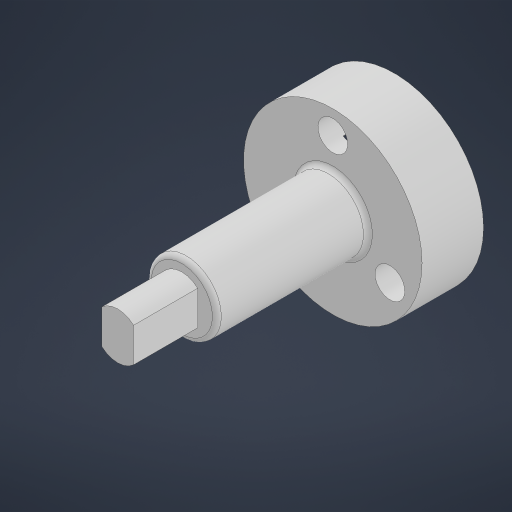
# Autodesk Inventor part: Mounting Adapter
Saved by Autodesk Inventor 2023 (Build 270158000, 158)
## iProperties
Created: 2023-03-26
Part Number: Mounting Adapter
Material: Generic
Document SubType Name: Modeling
Designer: Michael
Density: 1 g/cm^3
Appearance: Default
Author: Michael
Autodesk Inventor part; units mm, degrees
ref_plane "YZ Plane" through (0, 0, 0) normal (1, 0, 0) x (0, 1, 0)
ref_plane "XZ Plane" through (0, 0, 0) normal (0, 1, 0) x (-1, 0, 0)
ref_plane "XY Plane" through (0, 0, 0) normal (0, 0, 1) x (1, 0, 0)
sketch "Sketch1" plane through (0, 0, 0) normal (0, 0, 1) x (1, 0, 0)
  line L0 (6.5, 0) -> (19.5, 0) construction
  line L1 (0, 0) -> (13, 0)
  line L2 (13, 0) -> (6.5, 11.2583)
  line L3 (0, 0) -> (6.5, 11.2583)
  circle A0 centre (6.5, 3.7528) radius 6
  line L4 (6.5, 11.2583) -> (6.5, 0)
  circle A1 centre (6.5, 11.2583) radius 1.7
  circle A2 centre (13, 0) radius 1.7
  circle A3 centre (0, 0) radius 1.7
  circle A4 centre (6.5, 3.7528) radius 10.16
  point P0 (1.7, 0)
  point P1 (0.85, 1.4722)
  point P2 (0.9092, 1.5748)
  point P3 (5.5908, 9.6835)
  point P4 (5.65, 9.7861)
  point P5 (7.35, 9.7861)
  point P6 (7.4092, 9.6835)
  point P7 (12.0908, 1.5748)
  point P8 (12.15, 1.4722)
  point P9 (11.3, 0)
  point P10 (11.1815, 0)
  point P11 (1.8185, 0)
  dimension "d6" = 13
  dimension "d7" = 13
  dimension "d8" = 13
  dimension "d9" = 12
  dimension "d10" = 3.4
  dimension "d11" = 3.4
  dimension "d12" = 3.4
  dimension "d13" = 20.32
  constraints: 10 end point, 5 centre point, 4 coincident, 1 horizontal, 1 midpoint, 1 perpendicular, 1 point on line
  measures "d6" distance of L1.start L1.end
  measures "d7" distance of L1.end L2.end
  measures "d8" distance of L2.end L1.start
  measures "d9" diameter of A0
  measures "d10" diameter of A1
  measures "d11" diameter of A2
  measures "d12" diameter of A3
  measures "d13" diameter of A4
extrude "Extrusion1" add sketch "Sketch1" along normal blind 5
sketch "Sketch2" plane through (6.5, 3.7528, 5) normal (0, 0, 1) x (1, 0, 0)
  arc A0 (5.5908, -2.1779) -> (0.9092, 5.9307) centre (0, 0) ccw projected
  circle A1 centre (0, 0) radius 6
  circle A2 centre (0, 0) radius 3
  circle A3 centre (0, 0) radius 10.16 projected
  arc A4 (-5.65, -2.2805) -> (-4.8, -3.7528) centre (-6.5, -3.7528) ccw projected
  line L0 (-5.65, -2.2805) -> (-5.5908, -2.1779) projected
  arc A5 (-0.9092, 5.9307) -> (-5.5908, -2.1779) centre (0, 0) ccw projected
  line L1 (-0.9092, 5.9307) -> (-0.85, 6.0333) projected
  arc A6 (0.85, 6.0333) -> (-0.85, 6.0333) centre (0, 7.5056) ccw projected
  line L2 (0.85, 6.0333) -> (0.9092, 5.9307) projected
  arc A7 (5.5908, -2.1779) -> (0.9092, 5.9307) centre (0, 0) ccw projected
  line L3 (5.5908, -2.1779) -> (5.65, -2.2805) projected
  arc A8 (4.8, -3.7528) -> (5.65, -2.2805) centre (6.5, -3.7528) ccw projected
  line L4 (4.8, -3.7528) -> (4.6815, -3.7528) projected
  arc A9 (-4.6815, -3.7528) -> (4.6815, -3.7528) centre (0, 0) ccw projected
  line L5 (-4.6815, -3.7528) -> (-4.8, -3.7528) projected
  circle A10 centre (0, 7.5056) radius 1.7
  circle A11 centre (-6.5, -3.7528) radius 1.7
  circle A12 centre (6.5, -3.7528) radius 1.7
  point P0 (0.9092, 5.9307)
  point P1 (0.9092, 5.9307)
  point P2 (-4.6815, -3.7528)
  point P3 (-5.65, -2.2805)
  dimension "d16" = 6
  constraints: 5 coincident, 3 centre point, 6 other
  measures "d16" diameter of A2
extrude "Extrusion2" add sketch "Sketch2" along normal blind 2 contours A1 A12 A11 A10 A0 | L3 A12 A1 | A1 A10 L2 | A12 L4 A1 | A1 L1 A10 | L5 A11 A1 | A1 A11 L0 | A2 | A3
sketch "Sketch3" plane through (6.5, 3.7528, 7) normal (0, 0, 1) x (1, 0, 0)
  circle A0 centre (0, 0) radius 4
  point P0 (-6.5, -3.7528)
  dimension "d19" = 8
  constraints: 1 centre point
  measures "d19" diameter of A0
extrude "Extrusion3" add sketch "Sketch3" along normal blind 17
sketch "Sketch5" plane through (6.5, 3.7528, 24) normal (0, 0, 1) x (1, 0, 0)
  circle A0 centre (0, 0) radius 2
  point P0 (-6.5, -3.7528)
  dimension "d22" = 4
  constraints: 1 centre point
  measures "d22" diameter of A0
extrude "Extrusion4" cut sketch "Sketch5" against normal blind 22.6875
sketch "Sketch7" plane through (6.5, 3.7528, 24) normal (0, 0, 1) x (1, 0, 0)
  arc A0 (1.85, 1.9666) -> (-1.85, 1.9666) centre (0, 0) ccw
  line L0 (-1.85, 1.9666) -> (-1.85, -1.9666)
  arc A1 (-1.85, -1.9666) -> (1.85, -1.9666) centre (0, 0) ccw
  line L1 (1.85, -1.9666) -> (1.85, 1.9666)
  arc A2 (1.81, 1.9492) -> (-1.81, 1.9492) centre (0, 0) ccw
  line L2 (-1.81, 1.9492) -> (-1.81, -1.9492)
  arc A3 (-1.81, -1.9492) -> (1.81, -1.9492) centre (0, 0) ccw
  line L3 (1.81, -1.9492) -> (1.81, 1.9492)
  point P0 (-6.5, -3.7528)
  dimension "d30" = 0.04
  constraints: 8 end point, 8 point on circle, 4 centre point, 3 other
  measures "d30" distance between parallel lines of L1 L3
extrude "Extrusion5" add sketch "Sketch7" along normal blind 7.5 contours L3 A3 L2 A2
sketch "Sketch8" plane through (6.5, 3.7528, 24) normal (0, 0, 1) x (1, 0, 0)
  circle A0 centre (0, 0) radius 4 projected
  point P0 (-6.5, -3.7528)
extrude "Extrusion6" add sketch "Sketch8" along normal blind 0.2
fillet "Fillet1" radius 0.508 1 edges at (2.5, 3.7528, 7)
fillet "Fillet2" radius 0.508 1 edges at (2.5, 3.7528, 24.2)
body "Solid1"
